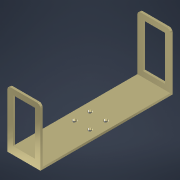
# Autodesk Inventor part: new-motor-base
Saved by Autodesk Inventor 2021 (Build 250183000, 183)
## iProperties
Created: 2021-02-13
Part Number: new-motor-base
Material: Generic
Document SubType Name: Modeling
Designer: vikki
Density: 1 g/cm^3
Appearance: Gold - Metal
Author: vikki
Autodesk Inventor part; units mm, degrees
ref_plane "YZ Plane" through (0, 0, 0) normal (1, 0, 0) x (0, 1, 0)
ref_plane "XZ Plane" through (0, 0, 0) normal (0, 1, 0) x (-1, 0, 0)
ref_plane "XY Plane" through (0, 0, 0) normal (0, 0, 1) x (1, 0, 0)
sketch "Sketch1" plane through (0, 0, 0) normal (0, 1, 0) x (-1, 0, 0)
  line L0 (-15, 60) -> (15, 60)
  line L1 (15, 60) -> (15, -60)
  line L2 (15, -60) -> (-15, -60)
  line L3 (-15, -60) -> (-15, 60)
  line L4 (-15, 60) -> (15, -60) construction
  line L5 (15, 60) -> (-15, -60) construction
  circle A0 centre (7.0711, -7.0711) radius 2
  line L6 (7.0711, -7.0711) -> (0, 0) construction
  circle A1 centre (0, 0) radius 65.2762 construction
  circle A2 centre (7.0711, 7.0711) radius 2
  circle A3 centre (-7.0711, 7.0711) radius 2
  circle A4 centre (-7.0711, -7.0711) radius 2
  dimension "d0" = 30
  dimension "d1" = 120
  dimension "d2" = 10
  dimension "d3" = 4
  dimension "d4" = 45
  dimension "d7" = 360
  constraints: 14 end point, 5 centre point, 2 midpoint, 2 parallel, 1 coincident, 1 horizontal, 1 perpendicular, 9 other
  measures "d0" distance of L1.end L2.end
  measures "d1" distance of L0.end L1.end
  measures "d2" distance of L6.end L6.start
  measures "d3" diameter of A0
  measures "d4" angle of L3 L6
extrude "Extrusion1" add sketch "Sketch1" along normal blind 2
sketch "Sketch2" plane through (0, 2, 0) normal (0, 1, 0) x (1, 0, 0)
  line L0 (15, 60) -> (-15, 60) projected
  line L1 (-15, 60) -> (15, 60)
  line L2 (15, 60) -> (15, 58)
  line L3 (15, 58) -> (-15, 58)
  line L4 (-15, 58) -> (-15, 60)
  line L5 (15, -60) -> (15, 60) projected
  point P0 (0, 0)
  dimension "d11" = 2
  constraints: 8 end point, 2 parallel, 1 collinear, 1 horizontal, 1 perpendicular
  measures "d11" distance of L1.end L2.end
extrude "Extrusion2" add sketch "Sketch2" along normal blind 60
sketch "Sketch3" plane through (15, 0, -60) normal (0, 0, -1) x (-1, 0, 0)
  line L0 (5, 54) -> (25, 54)
  line L1 (25, 54) -> (25, 14)
  line L2 (25, 14) -> (5, 14)
  line L3 (5, 14) -> (5, 54)
  line L4 (0, 0) -> (0, 62) projected
  line L5 (0, 62) -> (30, 62) projected
  point P0 (15, 0)
  dimension "d14" = 40
  dimension "d15" = 20
  dimension "d16" = 5
  dimension "d17" = 8
  constraints: 8 end point, 2 parallel, 1 horizontal, 1 perpendicular
  measures "d14" distance of L0.end L1.end
  measures "d15" distance of L1.end L2.end
  measures "d16" distance between parallel lines of L4 L3
  measures "d17" distance between parallel lines of L5 L0
extrude "Extrusion3" cut sketch "Sketch3" against normal up to surface (2 mm away)
fillet "Fillet1" radius 3 2 edges at (15, 62, -59) (-15, 62, -59)
mirror "Mirror1" about plane through (0, 0, 0) normal (0, 0, 1) of "Extrusion2", "Extrusion3", "Fillet1"
body "Solid1"
